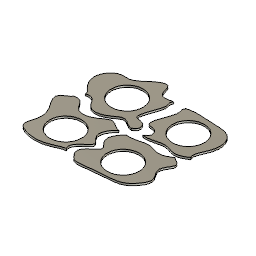
cnc_coasters (Autodesk Fusion 360 design; units mm, degrees)
Autodesk Fusion 360 part; units mm, degrees
sketch "Sketch1" plane through (0, 0, 0) normal (0, 0, 1) x (1, 0, 0)
  circle A0 centre (0, 0) radius 40
  circle A1 centre (-125, 0) radius 40
  circle A2 centre (-125, 125) radius 40
  circle A3 centre (-0.2384, 125.0002) radius 40
  spline S0 degree 5 poles (-207.6314, 63.7744) (-208.2849, 62.7401) (-209.3346, 60.6036) (-210.0647, 57.1888) (-209.2531, 52.2065) (-205.7445, 45.3105) (-200.6729, 37.8467) (-195.1473, 29.9518) (-190.1926, 21.7835) (-186.4596, 13.5031) (-184.2516, 5.2697) (-183.5868, -2.7645) (-184.2476, -10.4594) (-185.8359, -17.6919) (-187.8246, -24.3606) (-189.615, -30.3917) (-190.6186, -35.747) (-190.3352, -40.4318) (-188.4344, -44.5035) (-184.8287, -48.0774) (-179.6036, -51.2647) (-172.957, -54.1201) (-165.1299, -56.573) (-156.3596, -58.4047) (-146.8937, -59.3447) (-136.9919, -59.1458) (-126.9332, -57.6661) (-117.0215, -54.9522) (-107.5884, -51.311) (-99.0072, -47.417) (-91.623, -44.132) (-85.6726, -42.2787) (-81.2003, -42.4143) (-77.9914, -44.6392) (-75.4577, -48.3017) (-72.801, -52.3089) (-69.2415, -55.5762) (-64.2652, -57.5205) (-57.6631, -58.0952) (-49.4529, -57.5725) (-39.839, -56.4015) (-29.1566, -55.0455) (-17.8212, -53.8008) (-6.2846, -52.7699) (5.0028, -51.919) (15.6332, -51.109) (25.2785, -50.1361) (33.734, -48.7703) (40.9492, -46.792) (47.088, -44.0344) (52.4915, -40.4065) (57.5258, -35.8904) (62.4461, -30.5463) (67.2786, -24.5112) (71.6358, -18.0089) (74.8385, -11.3132) (76.2113, -4.6844) (75.3363, 1.688) (72.2998, 7.74) (68.0057, 13.6032) (63.8329, 19.5217) (61.173, 25.7397) (61.0235, 32.4035) (63.5265, 39.449) (67.6193, 46.5188) (71.6411, 53.1337) (73.888, 58.8508) (73.1348, 63.4112) (69.2968, 66.93) (63.5998, 69.9373) (57.7956, 73.1317) (53.6357, 77.2105) (52.138, 82.639) (53.292, 89.5484) (56.4475, 97.8307) (60.5474, 107.1912) (64.4323, 117.2178) (67.0934, 127.4413) (68, 137.405) (67.0595, 146.6957) (64.4635, 154.9645) (60.5723, 161.9498) (55.7809, 167.5007) (50.3992, 171.5978) (44.5095, 174.3817) (38.0397, 176.1054) (30.8618, 177.079) (22.8822, 177.6168) (14.1349, 177.9834) (4.8727, 178.3406) (-4.5218, 178.7604) (-13.6262, 179.239) (-22.0657, 179.7093) (-29.6044, 180.0541) (-36.2298, 180.1203) (-42.2541, 179.7292) (-48.1571, 178.7487) (-54.3939, 177.1789) (-61.2374, 175.2164) (-68.5546, 173.3668) (-75.7942, 172.3984) (-82.2773, 173.0694) (-87.421, 175.9018) (-90.9768, 180.9514) (-93.2963, 187.5417) (-95.1263, 194.5212) (-97.334, 200.597) (-100.6791, 204.6167) (-105.5147, 205.9289) (-111.705, 204.5065) (-118.8409, 200.7417) (-126.3854, 195.3211) (-133.8434, 189.0694) (-140.93, 182.8044) (-147.5411, 177.2519) (-153.7112, 172.9714) (-159.576, 170.2705) (-165.332, 169.1387) (-171.2009, 169.1384) (-177.3807, 169.4299) (-183.9775, 169.0296) (-190.9379, 167.0241) (-197.9893, 162.7873) (-204.5546, 156.2325) (-209.8847, 147.7189) (-213.2337, 137.891) (-214.0136, 127.5437) (-211.9707, 117.4719) (-207.323, 108.3388) (-200.9901, 100.5045) (-194.4129, 94.0254) (-189.1548, 88.747) (-186.5509, 84.3695) (-187.3781, 80.5208) (-191.4194, 76.8346) (-197.405, 73.0009) (-202.3697, 69.6134) (-205.4139, 66.8094) (-206.9779, 64.8087) (-207.6314, 63.7744) knots 0 0 0 0 0 0 0.00740741 0.01481481 0.02222222 0.02962963 0.03703704 0.04444444 0.05185185 0.05925926 0.06666667 0.07407407 0.08148148 0.08888889 0.0962963 0.1037037 0.11111111 0.11851852 0.12592593 0.13333333 0.14074074 0.14814815 0.15555556 0.16296296 0.17037037 0.17777778 0.18518519 0.19259259 0.2 0.20740741 0.21481481 0.22222222 0.22962963 0.23703704 0.24444444 0.25185185 0.25925926 0.26666667 0.27407407 0.28148148 0.28888889 0.2962963 0.3037037 0.31111111 0.31851852 0.32592593 0.33333333 0.34074074 0.34814815 0.35555556 0.36296296 0.37037037 0.37777778 0.38518519 0.39259259 0.4 0.40740741 0.41481481 0.42222222 0.42962963 0.43703704 0.44444444 0.45185185 0.45925926 0.46666667 0.47407407 0.48148148 0.48888889 0.4962963 0.5037037 0.51111111 0.51851852 0.52592593 0.53333333 0.54074074 0.54814815 0.55555556 0.56296296 0.57037037 0.57777778 0.58518519 0.59259259 0.6 0.60740741 0.61481481 0.62222222 0.62962963 0.63703704 0.64444444 0.65185185 0.65925926 0.66666667 0.67407407 0.68148148 0.68888889 0.6962963 0.7037037 0.71111111 0.71851852 0.72592593 0.73333333 0.74074074 0.74814815 0.75555556 0.76296296 0.77037037 0.77777778 0.78518519 0.79259259 0.8 0.80740741 0.81481481 0.82222222 0.82962963 0.83703704 0.84444444 0.85185185 0.85925926 0.86666667 0.87407407 0.88148148 0.88888889 0.8962963 0.9037037 0.91111111 0.91851852 0.92592593 0.93333333 0.94074074 0.94814815 0.95555556 0.96296296 0.97037037 0.97777778 0.98518519 0.99259259 1 1 1 1 1 1
  spline S1 degree 5 poles (-187.5043, 81.9947) (-186.0867, 82.3536) (-183.3482, 82.9263) (-179.5302, 83.3499) (-175.0197, 83.0431) (-170.3129, 81.2435) (-166.4231, 78.1485) (-163.1202, 74.0037) (-160.0071, 69.2327) (-156.6086, 64.3713) (-152.4827, 59.9841) (-147.3138, 56.5916) (-141.039, 54.5835) (-133.8711, 54.1714) (-126.1796, 55.3949) (-118.407, 58.1146) (-110.9707, 62.0081) (-104.1732, 66.5673) (-98.1015, 71.0856) (-92.6731, 74.7994) (-87.6912, 77.0387) (-82.8959, 77.3745) (-78.0166, 75.77) (-72.8242, 72.7287) (-67.1437, 69.0724) (-60.8683, 65.7211) (-53.9727, 63.4758) (-46.5279, 62.791) (-38.7124, 63.5771) (-30.7656, 65.3848) (-22.9459, 67.5607) (-15.4861, 69.4158) (-8.5525, 70.3811) (-2.1959, 70.1863) (3.6766, 68.9764) (9.2478, 67.158) (14.7462, 65.2801) (20.4016, 63.9115) (26.3923, 63.4972) (32.832, 64.3192) (39.7885, 66.5462) (45.7928, 69.5152) (50.5475, 72.4207) (53.8288, 74.6589) (55.4974, 75.8533) knots 0 0 0 0 0 0 0.025 0.05 0.075 0.1 0.125 0.15 0.175 0.2 0.225 0.25 0.275 0.3 0.325 0.35 0.375 0.4 0.425 0.45 0.475 0.5 0.525 0.55 0.575 0.6 0.625 0.65 0.675 0.7 0.725 0.75 0.775 0.8 0.825 0.85 0.875 0.9 0.925 0.95 0.975 1 1 1 1 1 1
  spline S2 degree 5 poles (-58.5037, 176.0113) (-58.8346, 175.2116) (-59.424, 173.6688) (-60.0909, 171.5244) (-60.5448, 169.0056) (-60.4351, 166.3665) (-59.7863, 164.072) (-58.8929, 161.7716) (-58.1898, 158.949) (-58.1024, 155.1037) (-58.9409, 149.8803) (-60.7478, 143.2526) (-63.3142, 135.5033) (-66.2691, 127.1143) (-69.1442, 118.6854) (-71.45, 110.8416) (-72.7443, 104.1473) (-72.7093, 99.0119) (-71.2142, 95.6117) (-68.4116, 93.7714) (-64.6977, 93.0123) (-60.5678, 92.7279) (-56.5127, 92.3124) (-52.8744, 91.332) (-49.812, 89.5865) (-47.3808, 87.0644) (-45.5774, 83.9216) (-44.4077, 80.4633) (-43.9119, 77.0789) (-44.1442, 74.0976) (-45.1624, 71.6806) (-47.0162, 69.6596) (-49.7182, 67.6206) (-53.2022, 65.0858) (-57.2925, 61.6505) (-61.6531, 57.1706) (-65.8328, 51.7472) (-69.346, 45.643) (-71.7417, 39.2201) (-72.676, 32.87) (-71.9871, 26.9455) (-69.7611, 21.6964) (-66.4248, 17.19) (-62.6453, 13.3419) (-59.1858, 9.9715) (-56.7724, 6.8496) (-55.9659, 3.7473) (-57.0077, 0.4902) (-59.7548, -3.0115) (-63.8083, -6.7891) (-68.5995, -10.8286) (-73.4961, -15.0903) (-77.8913, -19.5235) (-81.3197, -24.0869) (-83.4813, -28.754) (-84.1957, -33.5082) (-83.5397, -37.3749) (-82.3447, -40.3092) (-81.2357, -42.2806) (-80.6032, -43.2701) knots 0 0 0 0 0 0 0.018182 0.036364 0.054545 0.072727 0.090909 0.109091 0.127273 0.145455 0.163636 0.181818 0.2 0.218182 0.236364 0.254545 0.272727 0.290909 0.309091 0.327273 0.345455 0.363636 0.381818 0.4 0.418182 0.436364 0.454545 0.472727 0.490909 0.509091 0.527273 0.545455 0.563636 0.581818 0.6 0.618182 0.636364 0.654545 0.672727 0.690909 0.709091 0.727273 0.745455 0.763636 0.781818 0.8 0.818182 0.836364 0.854545 0.872727 0.890909 0.909091 0.927273 0.945455 0.963636 0.981818 1 1 1 1 1 1
  point P0 (-194.7196, 28.997)
  point P1 (-185.6055, -16.1937)
  point P2 (-190, -40)
  point P3 (-174.6335, -53.263)
  point P4 (-115.5178, -54.181)
  point P5 (-80.6032, -43.2701)
  point P6 (-71.4381, -53.3081)
  point P7 (-36.087, -55.9267)
  point P8 (37.6489, -47.5667)
  point P9 (64.2317, -28.1992)
  point P10 (74.4851, 2.5609)
  point P11 (61.5734, 31.8019)
  point P12 (72.9937, 61.6282)
  point P13 (55.4974, 75.8533)
  point P14 (64.9037, 119.8245)
  point P15 (55.0314, 167.6961)
  point P16 (22.7523, 177.5697)
  point P17 (-30, 180)
  point P18 (-58.5037, 176.0113)
  point P19 (-87.5064, 176.9006)
  point P20 (-99.4522, 202.6167)
  point P21 (-126.7931, 194.7816)
  point P22 (-163.2495, 169.7179)
  point P23 (-192.1108, 165.9203)
  point P24 (-209.9592, 114.2738)
  point P25 (-187.5043, 81.9947)
  point P26 (-166.1181, 77.4288)
  point P27 (-149.3521, 58.179)
  point P28 (-110.6316, 62.4676)
  point P29 (-82.9095, 76.8982)
  point P30 (-54.428, 63.9866)
  point P31 (-10, 70)
  point P32 (17.3455, 64.7461)
  point P33 (-60, 165)
  point P34 (-58.5037, 153.2288)
  point P35 (-71.8967, 97.7847)
  point P36 (-58.5037, 92.4681)
  point P37 (-46.4532, 85.2528)
  point P38 (-44.5544, 73.4804)
  point P39 (-54.428, 63.9866)
  point P40 (-71.291, 26.0167)
  point P41 (-56.4806, 4.7505)
  point P42 (-75.366, -17.0841)
  dimension "d1" = 80
  dimension "d2" = 80
  dimension "d3" = 80
  dimension "d4" = 80
  constraint coincident A0.centre origin
  constraint coincident P25 S1.start
  constraint coincident P13 S1.end
  constraint coincident P18 S2.start
  constraint coincident P39 P30
  constraint coincident P5 S2.end
  measures "d1" diameter of A0
  measures "d2" diameter of A1
  measures "d3" diameter of A2
  measures "d4" diameter of A3
extrude "Extrude1" add sketch "Sketch1" along normal blind 5 contours S0 S1 S2 picked at (-109.6829, 183.1488) makes body 1
extrude "Extrude2" add sketch "Sketch1" along normal blind 5 separate body contours S0 S1 S2 picked at (-56.6721, 129.1631) makes body 2
extrude "Extrude3" add sketch "Sketch1" along normal blind 5 separate body contours S0 S1 S2 picked at (-184.0328, 43.836) makes body 3
extrude "Extrude4" add sketch "Sketch1" along normal blind 5 separate body contours S0 S1 S2 picked at (43.1622, 43.696) makes body 4
move_body "Move1" bodies 1 to x (1, 0, 0) y (0, 1, 0) z (0, 0, 1) at (-10, 10, 0)
move_body "Move2" bodies 2 to x (1, 0, 0) y (0, 1, 0) z (0, 0, 1) at (20, 20, 0)
move_body "Move3" bodies 1 to x (1, 0, 0) y (0, 1, 0) z (0, 0, 1) at (0, 10, 0)
move_body "Move4" bodies 3 to x (1, 0, 0) y (0, 1, 0) z (0, 0, 1) at (-20, 0, 0)
sketch "Sketch2" plane through (0, 0, 5) normal (0, 0, 1) x (-1, 0, 0)
  circle A0 centre (135, -145) radius 40
  spline S0 degree 5 poles (197.5043, -101.9947) (196.0867, -102.3536) (193.3482, -102.9263) (189.5302, -103.3499) (185.0197, -103.0431) (180.3129, -101.2435) (176.4231, -98.1485) (173.1202, -94.0037) (170.0071, -89.2327) (166.6086, -84.3713) (162.4827, -79.9841) (157.3138, -76.5916) (151.039, -74.5835) (143.8711, -74.1714) (136.1796, -75.3949) (128.407, -78.1146) (120.9707, -82.0081) (114.1732, -86.5673) (108.1015, -91.0856) (102.6731, -94.7994) (97.6912, -97.0387) (92.8959, -97.3745) (88.0166, -95.77) (82.8242, -92.7287) (77.2379, -89.1331) (72.3313, -86.5026) (68.4137, -85.0049) (65.7331, -84.2748) (64.428, -83.9866) knots 0 0 0 0 0 0 0.025 0.05 0.075 0.1 0.125 0.15 0.175 0.2 0.225 0.25 0.275 0.3 0.325 0.35 0.375 0.4 0.425 0.45 0.475 0.5 0.525 0.55 0.575 0.597928 0.597928 0.597928 0.597928 0.597928 0.597928
  spline S1 degree 5 poles (64.428, -83.9866) (64.2087, -84.1689) (63.215, -84.9862) (61.522, -86.3101) (59.329, -87.9143) (57.0162, -89.6596) (55.1624, -91.6806) (54.1442, -94.0976) (53.9119, -97.0789) (54.4077, -100.4633) (55.5774, -103.9216) (57.3808, -107.0644) (59.812, -109.5865) (62.8744, -111.332) (66.5127, -112.3124) (70.5678, -112.7279) (74.6977, -113.0123) (78.4116, -113.7714) (81.2142, -115.6117) (82.7093, -119.0119) (82.7443, -124.1473) (81.45, -130.8416) (79.1442, -138.6854) (76.2691, -147.1143) (73.3142, -155.5033) (70.7478, -163.2526) (68.9409, -169.8803) (68.1024, -175.1037) (68.1898, -178.949) (68.8929, -181.7716) (69.7863, -184.072) (70.4351, -186.3665) (70.5448, -189.0056) (70.0909, -191.5244) (69.424, -193.6688) (68.8346, -195.2116) (68.5037, -196.0113) knots -0.568724 -0.568724 -0.568724 -0.568724 -0.568724 -0.568724 -0.563636 -0.545455 -0.527273 -0.509091 -0.490909 -0.472727 -0.454545 -0.436364 -0.418182 -0.4 -0.381818 -0.363636 -0.345455 -0.327273 -0.309091 -0.290909 -0.272727 -0.254545 -0.236364 -0.218182 -0.2 -0.181818 -0.163636 -0.145455 -0.127273 -0.109091 -0.090909 -0.072727 -0.054545 -0.036364 -0.018182 0 0 0 0 0 0
  spline S2 degree 5 poles (68.5037, -196.0113) (69.0653, -195.8585) (71.0142, -195.33) (74.4285, -194.4248) (79.41, -193.2524) (85.7942, -192.3984) (92.2773, -193.0694) (97.421, -195.9018) (100.9768, -200.9514) (103.2963, -207.5417) (105.1263, -214.5212) (107.334, -220.597) (110.6791, -224.6167) (115.5147, -225.9289) (121.705, -224.5065) (128.8409, -220.7417) (136.3854, -215.3211) (143.8434, -209.0694) (150.93, -202.8044) (157.5411, -197.2519) (163.7112, -192.9714) (169.576, -190.2705) (175.332, -189.1387) (181.2009, -189.1384) (187.3807, -189.4299) (193.9775, -189.0296) (200.9379, -187.0241) (207.9893, -182.7873) (214.5546, -176.2325) (219.8847, -167.7189) (223.2337, -157.891) (224.0136, -147.5437) (221.9707, -137.4719) (217.323, -128.3388) (210.9901, -120.5045) (204.4129, -114.0254) (199.5476, -109.1414) (197.4793, -105.9054) (197.1313, -103.7601) (197.3546, -102.4813) (197.5043, -101.9947) knots 0.70808 0.70808 0.70808 0.70808 0.70808 0.70808 0.711111 0.718519 0.725926 0.733333 0.740741 0.748148 0.755556 0.762963 0.77037 0.777778 0.785185 0.792593 0.8 0.807407 0.814815 0.822222 0.82963 0.837037 0.844444 0.851852 0.859259 0.866667 0.874074 0.881481 0.888889 0.896296 0.903704 0.911111 0.918519 0.925926 0.933333 0.940741 0.948148 0.955556 0.962963 0.967603 0.967603 0.967603 0.967603 0.967603 0.967603
  circle A1 centre (-19.7616, -145.0002) radius 40
  spline S3 degree 5 poles (38.5037, -196.0113) (38.8346, -195.2116) (39.424, -193.6688) (40.0909, -191.5244) (40.5448, -189.0056) (40.4351, -186.3665) (39.7863, -184.072) (38.8929, -181.7716) (38.1898, -178.949) (38.1024, -175.1037) (38.9409, -169.8803) (40.7478, -163.2526) (43.3142, -155.5033) (46.2691, -147.1143) (49.1442, -138.6854) (51.45, -130.8416) (52.7443, -124.1473) (52.7093, -119.0119) (51.2142, -115.6117) (48.4116, -113.7714) (44.6977, -113.0123) (40.5678, -112.7279) (36.5127, -112.3124) (32.8744, -111.332) (29.812, -109.5865) (27.3808, -107.0644) (25.5774, -103.9216) (24.4077, -100.4633) (23.9119, -97.0789) (24.1442, -94.0976) (25.1624, -91.6806) (27.0162, -89.6596) (29.329, -87.9143) (31.522, -86.3101) (33.215, -84.9862) (34.2087, -84.1689) (34.428, -83.9866) knots 0 0 0 0 0 0 0.018182 0.036364 0.054545 0.072727 0.090909 0.109091 0.127273 0.145455 0.163636 0.181818 0.2 0.218182 0.236364 0.254545 0.272727 0.290909 0.309091 0.327273 0.345455 0.363636 0.381818 0.4 0.418182 0.436364 0.454545 0.472727 0.490909 0.509091 0.527273 0.545455 0.563636 0.568724 0.568724 0.568724 0.568724 0.568724 0.568724
  spline S4 degree 5 poles (34.428, -83.9866) (34.31, -83.9606) (32.7666, -83.6268) (29.7371, -83.1495) (25.0944, -82.9351) (18.7124, -83.5771) (10.7656, -85.3848) (2.9459, -87.5607) (-4.5139, -89.4158) (-11.4475, -90.3811) (-17.8041, -90.1863) (-23.6766, -88.9764) (-29.2478, -87.158) (-34.7462, -85.2801) (-40.4016, -83.9115) (-46.3923, -83.4972) (-52.832, -84.3192) (-59.7885, -86.5462) (-65.7928, -89.5152) (-70.5475, -92.4207) (-73.8288, -94.6589) (-75.4974, -95.8533) knots 0.597928 0.597928 0.597928 0.597928 0.597928 0.597928 0.6 0.625 0.65 0.675 0.7 0.725 0.75 0.775 0.8 0.825 0.85 0.875 0.9 0.925 0.95 0.975 1 1 1 1 1 1
  spline S5 degree 5 poles (-75.4974, -95.8533) (-75.2241, -96.175) (-74.2739, -97.3903) (-73.0123, -99.6886) (-72.2829, -103.5066) (-73.292, -109.5484) (-76.4475, -117.8307) (-80.5474, -127.1912) (-84.4323, -137.2178) (-87.0934, -147.4413) (-88, -157.405) (-87.0595, -166.6957) (-84.4635, -174.9645) (-80.5723, -181.9498) (-75.7809, -187.5007) (-70.3992, -191.5978) (-64.5095, -194.3817) (-58.0397, -196.1054) (-50.8618, -197.079) (-42.8822, -197.6168) (-34.1349, -197.9834) (-24.8727, -198.3406) (-15.4782, -198.7604) (-6.3738, -199.239) (2.0657, -199.7093) (9.6044, -200.0541) (16.2298, -200.1203) (22.2541, -199.7292) (27.674, -198.829) (32.1284, -197.7449) (35.5334, -196.8219) (37.6928, -196.2318) (38.5037, -196.0113) knots 0.508354 0.508354 0.508354 0.508354 0.508354 0.508354 0.511111 0.518519 0.525926 0.533333 0.540741 0.548148 0.555556 0.562963 0.57037 0.577778 0.585185 0.592593 0.6 0.607407 0.614815 0.622222 0.62963 0.637037 0.644444 0.651852 0.659259 0.666667 0.674074 0.681481 0.688889 0.696296 0.703704 0.70808 0.70808 0.70808 0.70808 0.70808 0.70808
  circle A2 centre (0, 0) radius 40
  spline S6 degree 5 poles (54.428, -63.9866) (54.9922, -63.5174) (56.371, -62.3395) (58.652, -60.2494) (61.887, -56.867) (65.8328, -51.7472) (69.346, -45.643) (71.7417, -39.2201) (72.676, -32.87) (71.9871, -26.9455) (69.7611, -21.6964) (66.4248, -17.19) (62.6453, -13.3419) (59.1858, -9.9715) (56.7724, -6.8496) (55.9659, -3.7473) (57.0077, -0.4902) (59.7548, 3.0115) (63.8083, 6.7891) (68.5995, 10.8286) (73.4961, 15.0903) (77.8913, 19.5235) (81.3197, 24.0869) (83.4813, 28.754) (84.1957, 33.5082) (83.5397, 37.3749) (82.3447, 40.3092) (81.2357, 42.2806) (80.6032, 43.2701) knots 0.568724 0.568724 0.568724 0.568724 0.568724 0.568724 0.581818 0.6 0.618182 0.636364 0.654545 0.672727 0.690909 0.709091 0.727273 0.745455 0.763636 0.781818 0.8 0.818182 0.836364 0.854545 0.872727 0.890909 0.909091 0.927273 0.945455 0.963636 0.981818 1 1 1 1 1 1
  spline S7 degree 5 poles (80.6032, 43.2701) (80.0596, 43.5161) (78.8698, 44.2117) (77.2372, 45.7299) (75.3282, 48.4971) (72.801, 52.3089) (69.2415, 55.5762) (64.2652, 57.5205) (57.6631, 58.0952) (49.4529, 57.5725) (39.839, 56.4015) (29.1566, 55.0455) (17.8212, 53.8008) (6.2846, 52.7699) (-5.0028, 51.919) (-15.6332, 51.109) (-25.2785, 50.1361) (-33.734, 48.7703) (-40.9492, 46.792) (-47.088, 44.0344) (-52.4915, 40.4065) (-57.5258, 35.8904) (-62.4461, 30.5463) (-67.2786, 24.5112) (-71.6358, 18.0089) (-74.8385, 11.3132) (-76.2113, 4.6844) (-75.3363, -1.688) (-72.2998, -7.74) (-68.0057, -13.6032) (-63.8329, -19.5217) (-61.173, -25.7397) (-61.0235, -32.4035) (-63.5265, -39.449) (-67.6193, -46.5188) (-71.6411, -53.1337) (-73.888, -58.8508) (-73.1348, -63.4112) (-69.2968, -66.93) (-64.0239, -69.7134) (-59.8199, -72.0185) (-57.2674, -73.9637) (-55.9582, -75.3109) (-55.4974, -75.8533) knots 0.224028 0.224028 0.224028 0.224028 0.224028 0.224028 0.22963 0.237037 0.244444 0.251852 0.259259 0.266667 0.274074 0.281481 0.288889 0.296296 0.303704 0.311111 0.318519 0.325926 0.333333 0.340741 0.348148 0.355556 0.362963 0.37037 0.377778 0.385185 0.392593 0.4 0.407407 0.414815 0.422222 0.42963 0.437037 0.444444 0.451852 0.459259 0.466667 0.474074 0.481481 0.488889 0.496296 0.503704 0.508354 0.508354 0.508354 0.508354 0.508354 0.508354
  spline S8 degree 5 poles (-55.4974, -75.8533) (-53.8288, -74.6589) (-50.5475, -72.4207) (-45.7928, -69.5152) (-39.7885, -66.5462) (-32.832, -64.3192) (-26.3923, -63.4972) (-20.4016, -63.9115) (-14.7462, -65.2801) (-9.2478, -67.158) (-3.6766, -68.9764) (2.1959, -70.1863) (8.5525, -70.3811) (15.4861, -69.4158) (22.9459, -67.5607) (30.7656, -65.3848) (38.7124, -63.5771) (45.0944, -62.9351) (49.7371, -63.1495) (52.7666, -63.6268) (54.31, -63.9606) (54.428, -63.9866) knots -1 -1 -1 -1 -1 -1 -0.975 -0.95 -0.925 -0.9 -0.875 -0.85 -0.825 -0.8 -0.775 -0.75 -0.725 -0.7 -0.675 -0.65 -0.625 -0.6 -0.597928 -0.597928 -0.597928 -0.597928 -0.597928 -0.597928
  circle A3 centre (145, 0) radius 40
  spline S9 degree 5 poles (207.5043, -81.9947) (207.5935, -81.7046) (208.0048, -80.6454) (209.2371, -78.857) (212.1693, -76.3543) (217.405, -73.0009) (222.3697, -69.6134) (225.4139, -66.8094) (226.9779, -64.8087) (227.6314, -63.7744) (228.2849, -62.7401) (229.3346, -60.6036) (230.0647, -57.1888) (229.2531, -52.2065) (225.7445, -45.3105) (220.6729, -37.8467) (215.1473, -29.9518) (210.1926, -21.7835) (206.4596, -13.5031) (204.2516, -5.2697) (203.5868, 2.7645) (204.2476, 10.4594) (205.8359, 17.6919) (207.8246, 24.3606) (209.615, 30.3917) (210.6186, 35.747) (210.3352, 40.4318) (208.4344, 44.5035) (204.8287, 48.0774) (199.6036, 51.2647) (192.957, 54.1201) (185.1299, 56.573) (176.3596, 58.4047) (166.8937, 59.3447) (156.9919, 59.1458) (146.9332, 57.6661) (137.0215, 54.9522) (127.5884, 51.311) (119.0072, 47.417) (111.623, 44.132) (106.5725, 42.559) (103.4897, 42.403) (101.689, 42.8147) (100.7784, 43.1908) (100.6032, 43.2701) knots 0.967603 0.967603 0.967603 0.967603 0.967603 0.967603 0.97037 0.977778 0.985185 0.992593 1 1 1 1 1 1.007407 1.014815 1.022222 1.02963 1.037037 1.044444 1.051852 1.059259 1.066667 1.074074 1.081481 1.088889 1.096296 1.103704 1.111111 1.118519 1.125926 1.133333 1.140741 1.148148 1.155556 1.162963 1.17037 1.177778 1.185185 1.192593 1.2 1.207407 1.214815 1.222222 1.224028 1.224028 1.224028 1.224028 1.224028 1.224028
  spline S10 degree 5 poles (100.6032, 43.2701) (101.2357, 42.2806) (102.3447, 40.3092) (103.5397, 37.3749) (104.1957, 33.5082) (103.4813, 28.754) (101.3197, 24.0869) (97.8913, 19.5235) (93.4961, 15.0903) (88.5995, 10.8286) (83.8083, 6.7891) (79.7548, 3.0115) (77.0077, -0.4902) (75.9659, -3.7473) (76.7724, -6.8496) (79.1858, -9.9715) (82.6453, -13.3419) (86.4248, -17.19) (89.7611, -21.6964) (91.9871, -26.9455) (92.676, -32.87) (91.7417, -39.2201) (89.346, -45.643) (85.8328, -51.7472) (81.887, -56.867) (78.652, -60.2494) (76.371, -62.3395) (74.9922, -63.5174) (74.428, -63.9866) knots -1 -1 -1 -1 -1 -1 -0.981818 -0.963636 -0.945455 -0.927273 -0.909091 -0.890909 -0.872727 -0.854545 -0.836364 -0.818182 -0.8 -0.781818 -0.763636 -0.745455 -0.727273 -0.709091 -0.690909 -0.672727 -0.654545 -0.636364 -0.618182 -0.6 -0.581818 -0.568724 -0.568724 -0.568724 -0.568724 -0.568724 -0.568724
  spline S11 degree 5 poles (74.428, -63.9866) (75.7331, -64.2748) (78.4137, -65.0049) (82.3313, -66.5026) (87.2379, -69.1331) (92.8242, -72.7287) (98.0166, -75.77) (102.8959, -77.3745) (107.6912, -77.0387) (112.6731, -74.7994) (118.1015, -71.0856) (124.1732, -66.5673) (130.9707, -62.0081) (138.407, -58.1146) (146.1796, -55.3949) (153.8711, -54.1714) (161.039, -54.5835) (167.3138, -56.5916) (172.4827, -59.9841) (176.6086, -64.3713) (180.0071, -69.2327) (183.1202, -74.0037) (186.4231, -78.1485) (190.3129, -81.2435) (195.0197, -83.0431) (199.5302, -83.3499) (203.3482, -82.9263) (206.0867, -82.3536) (207.5043, -81.9947) knots -0.597928 -0.597928 -0.597928 -0.597928 -0.597928 -0.597928 -0.575 -0.55 -0.525 -0.5 -0.475 -0.45 -0.425 -0.4 -0.375 -0.35 -0.325 -0.3 -0.275 -0.25 -0.225 -0.2 -0.175 -0.15 -0.125 -0.1 -0.075 -0.05 -0.025 0 0 0 0 0 0
